Autodesk Inventor part; units mm, degrees
(part 2 of 2)
sketch "スケッチ15" plane through (0, 0, -5) normal (0, 0, -1) x (-1, 0, 0)
  line L0 (-98.885049, -17.626881) -> (-98.885049, -29.356351)
  arc A0 (-98.885049, -29.356351) -> (-98.708578, -29.923625) centre (-97.885049, -29.356351) ccw
  arc A1 (-96.237392, -35.660714) -> (-98.708578, -29.923625) centre (-111.885049, -39.000002) ccw
  arc A2 (-96.237392, -35.660714) -> (-94.615037, -36.216716) centre (-95.259414, -35.452009) ccw
  line L1 (-94.615037, -36.216716) -> (-87.366936, -30.109143)
  arc A3 (-87.366936, -30.109143) -> (-87.246605, -28.700058) centre (-88.011313, -29.344435) ccw
  line L2 (-87.246605, -28.700058) -> (-97.120341, -16.982504)
  arc A4 (-97.120341, -16.982504) -> (-98.885049, -17.626881) centre (-97.885049, -17.626881) ccw
  line L3 (-95.269293, -14.523557) -> (-84.952482, -26.766926)
  arc A5 (-84.952482, -26.766926) -> (-83.543397, -26.887257) centre (-84.187774, -26.122549) ccw
  line L4 (-83.543397, -26.887257) -> (-68.236506, -13.988985)
  arc A6 (-68.236506, -13.988985) -> (-68.451315, -12.321243) centre (-68.880883, -13.224277) ccw
  arc A7 (-70.985635, -10.277156) -> (-68.451315, -12.321243) centre (-65.444342, -6) ccw
  arc A8 (-70.985635, -10.277156) -> (-71.610635, -9.902156) centre (-71.777249, -10.888178) ccw
  arc A9 (-73.833202, -9.125) -> (-71.610635, -9.902156) centre (-70.444342, -3) ccw
  arc A10 (-73.833202, -9.125) -> (-74.317325, -9) centre (-74.317325, -10) ccw
  line L5 (-74.317325, -9) -> (-80.016712, -9)
  arc A11 (-80.016712, -9) -> (-80.500835, -9.125) centre (-80.016712, -10) ccw
  arc A12 (-82.723402, -9.902156) -> (-80.500835, -9.125) centre (-83.889695, -3) ccw
  arc A13 (-82.723402, -9.902156) -> (-83.348402, -10.277156) centre (-82.556788, -10.888178) ccw
  arc A14 (-91.952195, -12.294529) -> (-83.348402, -10.277156) centre (-88.889695, -6) ccw
  arc A15 (-91.952195, -12.294529) -> (-92.827195, -12.294529) centre (-92.389695, -13.193747) ccw
  arc A16 (-94.677724, -12.894282) -> (-92.827195, -12.294529) centre (-95.889695, -6) ccw
  arc A17 (-94.677724, -12.894282) -> (-95.269293, -14.523557) centre (-94.504585, -13.87918) ccw
  line L6 (-57.444342, -3) -> (-54.444342, -3)
  arc A18 (-54.444342, -3) -> (-52.444342, -3) centre (-53.444342, -3) ccw
  line L7 (-52.444342, -3) -> (-49.444342, -3)
  line L8 (-49.444342, -3) -> (-49.444342, -6)
  line L9 (-49.444342, -6) -> (-102.219392, -50.47062)
  arc A19 (-121.057661, -50.868582) -> (-102.219392, -50.47062) centre (-111.885049, -39.000002) ccw
  line L10 (-121.057661, -50.868582) -> (-127.651316, -45.772687)
  line L11 (-127.651316, -45.772687) -> (-119.12697, -45.895985)
  arc A20 (-119.12697, -45.895985) -> (-104.885049, -31.858573) centre (-111.885049, -39.000002) ccw
  line L12 (-104.885049, -31.858573) -> (-104.885049, -3)
  line L13 (-104.885049, -3) -> (-101.889695, -3)
  arc A21 (-101.889695, -3) -> (-99.889695, -3) centre (-100.889695, -3) ccw
  line L14 (-99.889695, -3) -> (-96.889695, -3)
  line L15 (-96.889695, -3) -> (-96.889695, -6)
  arc A22 (-96.889695, -6) -> (-94.889695, -6) centre (-95.889695, -6) ccw
  line L16 (-94.889695, -6) -> (-89.889695, -6)
  arc A23 (-89.889695, -6) -> (-87.889695, -6) centre (-88.889695, -6) ccw
  line L17 (-87.889695, -6) -> (-87.889695, -3)
  line L18 (-87.889695, -3) -> (-84.889695, -3)
  arc A24 (-84.889695, -3) -> (-82.889695, -3) centre (-83.889695, -3) ccw
  line L19 (-82.889695, -3) -> (-71.444342, -3)
  arc A25 (-71.444342, -3) -> (-69.444342, -3) centre (-70.444342, -3) ccw
  line L20 (-69.444342, -3) -> (-66.444342, -3)
  line L21 (-66.444342, -3) -> (-66.444342, -6)
  arc A26 (-66.444342, -6) -> (-64.444342, -6) centre (-65.444342, -6) ccw
  line L22 (-64.444342, -6) -> (-59.444342, -6)
  arc A27 (-59.444342, -6) -> (-57.444342, -6) centre (-58.444342, -6) ccw
  line L23 (-57.444342, -6) -> (-57.444342, -3)
  line L24 (-107.885049, -23.783101) -> (-107.885049, -15.626145)
  arc A28 (-107.885049, -15.626145) -> (-109.702802, -15.050577) centre (-108.885049, -15.626145) ccw
  line L25 (-109.702802, -15.050577) -> (-113.542064, -20.505302)
  arc A29 (-113.542064, -20.505302) -> (-113.299879, -21.898624) centre (-112.72431, -21.08087) ccw
  line L26 (-113.299879, -21.898624) -> (-109.460618, -24.600855)
  arc A30 (-109.460618, -24.600855) -> (-107.885049, -23.783101) centre (-108.885049, -23.783101) ccw
  arc A31 (-123.011027, -34.504158) -> (-123.823452, -37.785703) centre (-111.885049, -39.000002) ccw
  line L27 (-123.823452, -37.785703) -> (-124.225152, -41.735024)
  arc A32 (-124.225152, -41.735024) -> (-123.244748, -42.836111) centre (-123.230285, -41.836215) ccw
  line L28 (-123.244748, -42.836111) -> (-120.427294, -42.876863)
  arc A33 (-120.427294, -42.876863) -> (-119.4653, -41.557305) centre (-120.412831, -41.876968) ccw
  arc A34 (-119.448659, -36.393892) -> (-119.4653, -41.557305) centre (-111.885049, -39.000002) ccw
  arc A35 (-119.448659, -36.393892) -> (-119.818541, -35.250375) centre (-120.39411, -36.068129) ccw
  line L29 (-119.818541, -35.250375) -> (-121.508293, -34.061058)
  arc A36 (-121.508293, -34.061058) -> (-123.011027, -34.504158) centre (-122.083862, -34.878811) ccw
  line L30 (-108.30948, -29.07966) -> (-115.026585, -24.351884)
  arc A37 (-115.026585, -24.351884) -> (-116.419907, -24.594069) centre (-115.602154, -25.169638) ccw
  line L31 (-116.419907, -24.594069) -> (-120.259168, -30.048794)
  arc A38 (-120.259168, -30.048794) -> (-120.016984, -31.442116) centre (-119.441415, -30.624363) ccw
  line L32 (-120.016984, -31.442116) -> (-118.091835, -32.797115)
  arc A39 (-118.091835, -32.797115) -> (-116.890576, -32.759433) centre (-117.516266, -31.979362) ccw
  arc A40 (-109.218382, -31.45753) -> (-116.890576, -32.759433) centre (-111.885049, -39.000002) ccw
  arc A41 (-109.218382, -31.45753) -> (-107.885049, -30.514721) centre (-108.885049, -30.514721) ccw
  line L33 (-107.885049, -30.514721) -> (-107.885049, -29.897414)
  arc A42 (-107.885049, -29.897414) -> (-108.30948, -29.07966) centre (-108.885049, -29.897414) ccw
  circle A43 centre (-111.885049, -39.000002) radius 3
  line L34 (-104.885049, -3) -> (-104.889695, -3)
  line L35 (-104.885049, -31.858573) -> (-104.885049, -3)
  arc A44 (-119.12697, -45.895985) -> (-104.885049, -31.858573) centre (-111.885049, -39.000002) ccw
  line L36 (-127.651316, -45.772687) -> (-119.12697, -45.895985)
  line L37 (-126.808053, -37.482129) -> (-127.651316, -45.772687)
  arc A45 (-124.15135, -30.366471) -> (-126.808053, -37.482129) centre (-111.885049, -39.000002) ccw
  line L38 (-104.889695, -3) -> (-124.15135, -30.366471)
  point P0 (0, 0)
  point P1 (0, 0)
  constraints: 90 point on circle, 78 end point, 46 centre point, 11 horizontal, 10 vertical, 194 other
extrude "押し出し17" cut sketch "スケッチ15" against normal blind 4 contours A4 L2 A3 L1 A2 A1 A0 L0 | A17 A16 A15 A14 A13 A12 A11 L5 A10 A9 A8 A7 A6 L4 A5 L3 | A30 L26 A29 L25 A28 L24 | A36 L29 A35 A34 A33 L28 A32 L27 A31 | A42 L33 A41 A40 A39 L32 A38 L31 A37 L30
sketch "スケッチ16" plane through (0, 0, -5) normal (0, 0, -1) x (-1, 0, 0)
  arc A0 (-82.723402, -9.902156) -> (-80.500835, -9.125) centre (-83.889695, -3) ccw
  arc A1 (-82.723402, -9.902156) -> (-83.348402, -10.277156) centre (-82.556788, -10.888178) ccw
  arc A2 (-91.952195, -12.294529) -> (-83.348402, -10.277156) centre (-88.889695, -6) ccw
  arc A3 (-91.952195, -12.294529) -> (-92.827195, -12.294529) centre (-92.389695, -13.193747) ccw
  arc A4 (-94.677724, -12.894282) -> (-92.827195, -12.294529) centre (-95.889695, -6) ccw
  arc A5 (-94.677724, -12.894282) -> (-95.269293, -14.523557) centre (-94.504585, -13.87918) ccw
  line L0 (-95.269293, -14.523557) -> (-84.952482, -26.766926)
  arc A6 (-84.952482, -26.766926) -> (-83.543397, -26.887257) centre (-84.187774, -26.122549) ccw
  line L1 (-83.543397, -26.887257) -> (-68.236506, -13.988985)
  arc A7 (-68.236506, -13.988985) -> (-68.451315, -12.321243) centre (-68.880883, -13.224277) ccw
  arc A8 (-70.985635, -10.277156) -> (-68.451315, -12.321243) centre (-65.444342, -6) ccw
  arc A9 (-70.985635, -10.277156) -> (-71.610635, -9.902156) centre (-71.777249, -10.888178) ccw
  arc A10 (-73.833202, -9.125) -> (-71.610635, -9.902156) centre (-70.444342, -3) ccw
  arc A11 (-73.833202, -9.125) -> (-74.317325, -9) centre (-74.317325, -10) ccw
  line L2 (-74.317325, -9) -> (-80.016712, -9)
  arc A12 (-80.016712, -9) -> (-80.500835, -9.125) centre (-80.016712, -10) ccw
  line L3 (-94.615037, -36.216716) -> (-87.366936, -30.109143)
  arc A13 (-87.366936, -30.109143) -> (-87.246605, -28.700058) centre (-88.011313, -29.344435) ccw
  line L4 (-87.246605, -28.700058) -> (-97.120341, -16.982504)
  arc A14 (-97.120341, -16.982504) -> (-98.885049, -17.626881) centre (-97.885049, -17.626881) ccw
  line L5 (-98.885049, -17.626881) -> (-98.885049, -29.356351)
  arc A15 (-98.885049, -29.356351) -> (-98.708578, -29.923625) centre (-97.885049, -29.356351) ccw
  arc A16 (-96.237392, -35.660714) -> (-98.708578, -29.923625) centre (-111.885049, -39.000002) ccw
  arc A17 (-96.237392, -35.660714) -> (-94.615037, -36.216716) centre (-95.259414, -35.452009) ccw
  line L6 (-127.651316, -45.772687) -> (-119.12697, -45.895985)
  arc A18 (-119.12697, -45.895985) -> (-104.885049, -31.858573) centre (-111.885049, -39.000002) ccw
  line L7 (-104.885049, -31.858573) -> (-104.885049, -3)
  line L8 (-104.885049, -3) -> (-101.889695, -3)
  arc A19 (-101.889695, -3) -> (-99.889695, -3) centre (-100.889695, -3) ccw
  line L9 (-99.889695, -3) -> (-96.889695, -3)
  line L10 (-96.889695, -3) -> (-96.889695, -6)
  arc A20 (-96.889695, -6) -> (-94.889695, -6) centre (-95.889695, -6) ccw
  line L11 (-94.889695, -6) -> (-89.889695, -6)
  arc A21 (-89.889695, -6) -> (-87.889695, -6) centre (-88.889695, -6) ccw
  line L12 (-87.889695, -6) -> (-87.889695, -3)
  line L13 (-87.889695, -3) -> (-84.889695, -3)
  arc A22 (-84.889695, -3) -> (-82.889695, -3) centre (-83.889695, -3) ccw
  line L14 (-82.889695, -3) -> (-71.444342, -3)
  arc A23 (-71.444342, -3) -> (-69.444342, -3) centre (-70.444342, -3) ccw
  line L15 (-69.444342, -3) -> (-66.444342, -3)
  line L16 (-66.444342, -3) -> (-66.444342, -6)
  arc A24 (-66.444342, -6) -> (-64.444342, -6) centre (-65.444342, -6) ccw
  line L17 (-64.444342, -6) -> (-59.444342, -6)
  arc A25 (-59.444342, -6) -> (-57.444342, -6) centre (-58.444342, -6) ccw
  line L18 (-57.444342, -6) -> (-57.444342, -3)
  line L19 (-57.444342, -3) -> (-54.444342, -3)
  arc A26 (-54.444342, -3) -> (-52.444342, -3) centre (-53.444342, -3) ccw
  line L20 (-52.444342, -3) -> (-49.444342, -3)
  line L21 (-49.444342, -3) -> (-49.444342, -6)
  line L22 (-49.444342, -6) -> (-102.219392, -50.47062)
  arc A27 (-121.057661, -50.868582) -> (-102.219392, -50.47062) centre (-111.885049, -39.000002) ccw
  line L23 (-121.057661, -50.868582) -> (-127.651316, -45.772687)
  line L24 (-84.889695, 0.872983) -> (-84.889695, -6)
  arc A28 (-91.535447, -9) -> (-84.889695, -6) centre (-88.889695, -6) ccw
  line L25 (-91.535447, -9) -> (-93.243944, -9)
  arc A29 (-99.889695, -6) -> (-93.243944, -9) centre (-95.889695, -6) ccw
  line L26 (-99.889695, -6) -> (-99.889695, 0.872983)
  arc A30 (-101.885049, 0.87418) -> (-99.889695, 0.872983) centre (-100.889695, -3) ccw
  line L27 (-101.885049, 0.87418) -> (-101.885049, -30.693378)
  arc A31 (-120.335431, -48.878819) -> (-101.885049, -30.693378) centre (-111.885049, -39.000002) ccw
  line L28 (-120.335431, -48.878819) -> (-118.695646, -48.902538)
  line L29 (-118.695646, -48.902538) -> (-119.223138, -48.494866)
  arc A32 (-119.223138, -48.494866) -> (-104.152524, -48.176497) centre (-111.885049, -39.000002) ccw
  line L30 (-104.152524, -48.176497) -> (-52.444342, -4.604868)
  line L31 (-52.444342, -4.604868) -> (-52.444342, 0.872983)
  arc A33 (-54.444342, 0.872983) -> (-52.444342, 0.872983) centre (-53.444342, -3) ccw
  line L32 (-54.444342, 0.872983) -> (-54.444342, -6)
  arc A34 (-61.090093, -9) -> (-54.444342, -6) centre (-58.444342, -6) ccw
  line L33 (-61.090093, -9) -> (-62.79859, -9)
  arc A35 (-69.444342, -6) -> (-62.79859, -9) centre (-65.444342, -6) ccw
  line L34 (-69.444342, -6) -> (-69.444342, 0.872983)
  arc A36 (-73.090093, -6) -> (-69.444342, 0.872983) centre (-70.444342, -3) ccw
  line L35 (-73.090093, -6) -> (-81.243944, -6)
  arc A37 (-84.889695, 0.872983) -> (-81.243944, -6) centre (-83.889695, -3) ccw
  line L36 (-87.366936, -30.109143) -> (-94.615037, -36.216716)
  line L37 (-94.615037, -36.216716) -> (-98.912059, -39.83758)
  line L38 (-98.885049, -29.356351) -> (-98.885049, -17.626881)
  line L39 (-98.885049, -29.356351) -> (-98.885049, -39.000002)
  line L40 (-87.366936, -30.109143) -> (-94.615037, -36.216716)
  line L41 (-68.236506, -13.988985) -> (-83.543397, -26.887257)
  line L42 (-68.236506, -13.988985) -> (-62.315879, -9)
  arc A38 (-94.677724, -12.894282) -> (-95.269293, -14.523557) centre (-94.504585, -13.87918) ccw
  line L43 (-95.269293, -14.523557) -> (-101.885049, -6.672377)
  line L44 (-98.885049, -17.626881) -> (-98.885049, -6.461415)
  point P0 (0, 0)
  point P1 (-84.980691, -6.848341)
  point P2 (-98.885049, -8.65101)
  point P3 (-98.885049, -10.232596)
  point P4 (-69.353346, -6.848341)
  dimension "d151" = 3
  constraints: 34 end point, 23 point on circle, 10 centre point, 5 collinear, 2 point on line, 21 other
  measures "d151" distance between parallel lines of L14 L35
extrude "押し出し18" cut sketch "スケッチ16" against normal blind 4 contours A1 A2 A3 A4 A5 L43 L44 A29 L25 A28 A37 L35 A36 A35 L33 L42 A7 A8 A9 A10 A11 L2 A12 A0 | A15 A16 A17 L37 A31 L39
fillet "フィレット3" radius 1 11 edges at (62.3159, -9, -3) (62.7986, -9, -3) (69.3533, -6.8483, -3) (73.0901, -6, -3) (81.2439, -6, -3) (84.9807, -6.8483, -3) (91.5354, -9, -3) (93.2439, -9, -3) (98.885, -8.651, -3) (98.885, -10.2326, -3) (98.9121, -39.8376, -3)
sketch "スケッチ17" plane through (0, 0, -5) normal (0, 0, -1) x (-1, 0, 0)
  arc A0 (-98.885049, -37.664486) -> (-97.240672, -38.429194) centre (-97.885049, -37.664486) ccw
  line L0 (-97.240672, -38.429194) -> (-87.366936, -30.109143)
  arc A1 (-87.366936, -30.109143) -> (-87.246605, -28.700058) centre (-88.011313, -29.344435) ccw
  line L1 (-87.246605, -28.700058) -> (-97.120341, -16.982504)
  arc A2 (-97.120341, -16.982504) -> (-98.885049, -17.626881) centre (-97.885049, -17.626881) ccw
  line L2 (-98.885049, -17.626881) -> (-98.885049, -37.664486)
  arc A3 (-96.813663, -9.891823) -> (-97.809362, -11.509155) centre (-97.044655, -10.864778) ccw
  line L3 (-97.809362, -11.509155) -> (-84.952482, -26.766926)
  arc A4 (-84.952482, -26.766926) -> (-83.543397, -26.887257) centre (-84.187774, -26.122549) ccw
  line L4 (-83.543397, -26.887257) -> (-65.532789, -11.710713)
  arc A5 (-65.532789, -11.710713) -> (-66.030602, -9.956804) centre (-66.177167, -10.946005) ccw
  arc A6 (-69.116255, -7.586522) -> (-66.030602, -9.956804) centre (-65.444342, -6) ccw
  arc A7 (-69.116255, -7.586522) -> (-70.116255, -6.986522) centre (-70.034233, -7.983153) ccw
  arc A8 (-72.844342, -6.2) -> (-70.116255, -6.986522) centre (-70.444342, -3) ccw
  arc A9 (-72.844342, -6.2) -> (-73.444342, -6) centre (-73.444342, -7) ccw
  line L5 (-73.444342, -6) -> (-80.889695, -6)
  arc A10 (-80.889695, -6) -> (-81.489695, -6.2) centre (-80.889695, -7) ccw
  arc A11 (-84.217782, -6.986522) -> (-81.489695, -6.2) centre (-83.889695, -3) ccw
  arc A12 (-84.217782, -6.986522) -> (-85.217782, -7.586522) centre (-84.299804, -7.983153) ccw
  arc A13 (-91.289695, -9.2) -> (-85.217782, -7.586522) centre (-88.889695, -6) ccw
  arc A14 (-91.289695, -9.2) -> (-91.889695, -9) centre (-91.889695, -10) ccw
  line L6 (-91.889695, -9) -> (-92.889695, -9)
  arc A15 (-92.889695, -9) -> (-93.489695, -9.2) centre (-92.889695, -10) ccw
  arc A16 (-96.813663, -9.891823) -> (-93.489695, -9.2) centre (-95.889695, -6) ccw
  line L7 (-127.651316, -45.772687) -> (-119.12697, -45.895985)
  arc A17 (-119.12697, -45.895985) -> (-104.885049, -31.858573) centre (-111.885049, -39.000002) ccw
  line L8 (-104.885049, -31.858573) -> (-104.885049, -3)
  line L9 (-104.885049, -3) -> (-101.889695, -3)
  arc A18 (-101.889695, -3) -> (-99.889695, -3) centre (-100.889695, -3) ccw
  line L10 (-99.889695, -3) -> (-96.889695, -3)
  line L11 (-96.889695, -3) -> (-96.889695, -6)
  arc A19 (-96.889695, -6) -> (-94.889695, -6) centre (-95.889695, -6) ccw
  line L12 (-94.889695, -6) -> (-89.889695, -6)
  arc A20 (-89.889695, -6) -> (-87.889695, -6) centre (-88.889695, -6) ccw
  line L13 (-87.889695, -6) -> (-87.889695, -3)
  line L14 (-87.889695, -3) -> (-84.889695, -3)
  arc A21 (-84.889695, -3) -> (-82.889695, -3) centre (-83.889695, -3) ccw
  line L15 (-82.889695, -3) -> (-71.444342, -3)
  arc A22 (-71.444342, -3) -> (-69.444342, -3) centre (-70.444342, -3) ccw
  line L16 (-69.444342, -3) -> (-66.444342, -3)
  line L17 (-66.444342, -3) -> (-66.444342, -6)
  arc A23 (-66.444342, -6) -> (-64.444342, -6) centre (-65.444342, -6) ccw
  line L18 (-64.444342, -6) -> (-59.444342, -6)
  arc A24 (-59.444342, -6) -> (-57.444342, -6) centre (-58.444342, -6) ccw
  line L19 (-57.444342, -6) -> (-57.444342, -3)
  line L20 (-57.444342, -3) -> (-54.444342, -3)
  arc A25 (-54.444342, -3) -> (-52.444342, -3) centre (-53.444342, -3) ccw
  line L21 (-52.444342, -3) -> (-49.444342, -3)
  line L22 (-49.444342, -3) -> (-49.444342, -6)
  line L23 (-49.444342, -6) -> (-102.219392, -50.47062)
  arc A26 (-121.057661, -50.868582) -> (-102.219392, -50.47062) centre (-111.885049, -39.000002) ccw
  line L24 (-121.057661, -50.868582) -> (-127.651316, -45.772687)
  line L25 (-104.796901, -47.411789) -> (-60.016711, -9.677996)
  line L26 (-70.444342, -6) -> (-70.444342, 2)
  arc A27 (-73.444342, -7) -> (-70.444342, 2) centre (-70.444342, -3) ccw
  line L27 (-73.444342, -7) -> (-80.889695, -7)
  arc A28 (-83.889695, 2) -> (-80.889695, -7) centre (-83.889695, -3) ccw
  line L28 (-83.889695, 2) -> (-83.889695, -6)
  arc A29 (-91.889695, -10) -> (-83.889695, -6) centre (-88.889695, -6) ccw
  line L29 (-91.889695, -10) -> (-92.889695, -10)
  arc A30 (-100.885049, -6.215503) -> (-92.889695, -10) centre (-95.889695, -6) ccw
  line L30 (-100.885049, -6.215503) -> (-100.885049, -32.071799)
  line L31 (-61.090093, -9) -> (-62.79859, -9)
  arc A31 (-69.444342, -6) -> (-62.79859, -9) centre (-65.444342, -6) ccw
  line L32 (-69.444342, -6) -> (-69.444342, -6)
  line L33 (-69.444342, -6) -> (-67.79859, -6)
  arc A32 (-73.090093, -6) -> (-67.79859, -6) centre (-70.444342, -3) ccw
  line L34 (-73.090093, -6) -> (-81.243944, -6)
  arc A33 (-86.535447, -6) -> (-81.243944, -6) centre (-83.889695, -3) ccw
  line L35 (-86.535447, -6) -> (-84.889695, -6)
  line L36 (-84.889695, -6) -> (-84.889695, -6)
  arc A34 (-91.535447, -9) -> (-84.889695, -6) centre (-88.889695, -6) ccw
  line L37 (-91.535447, -9) -> (-93.243944, -9)
  arc A35 (-99.889695, -6) -> (-93.243944, -9) centre (-95.889695, -6) ccw
  line L38 (-99.889695, -6) -> (-99.889695, -6)
  line L39 (-99.889695, -6) -> (-98.243944, -6)
  arc A36 (-103.535447, -6) -> (-98.243944, -6) centre (-100.889695, -3) ccw
  line L40 (-103.535447, -6) -> (-101.885049, -6)
  line L41 (-101.885049, -6) -> (-101.885049, -30.693378)
  arc A37 (-120.335431, -48.878819) -> (-101.885049, -30.693378) centre (-111.885049, -39.000002) ccw
  line L42 (-120.335431, -48.878819) -> (-118.695646, -48.902538)
  line L43 (-118.695646, -48.902538) -> (-119.223138, -48.494866)
  arc A38 (-119.223138, -48.494866) -> (-104.152524, -48.176497) centre (-111.885049, -39.000002) ccw
  line L44 (-104.152524, -48.176497) -> (-52.444342, -4.604868)
  line L45 (-52.444342, -4.604868) -> (-52.444342, -6)
  line L46 (-52.444342, -6) -> (-50.79859, -6)
  arc A39 (-56.090093, -6) -> (-50.79859, -6) centre (-53.444342, -3) ccw
  line L47 (-56.090093, -6) -> (-54.444342, -6)
  line L48 (-54.444342, -6) -> (-54.444342, -6)
  arc A40 (-61.090093, -9) -> (-54.444342, -6) centre (-58.444342, -6) ccw
  line L49 (-84.952482, -26.766926) -> (-97.809362, -11.509155)
  line L50 (-84.952482, -26.766926) -> (-76.330152, -36.999387)
  arc A41 (-87.366936, -30.109143) -> (-87.246605, -28.700058) centre (-88.011313, -29.344435) ccw
  line L51 (-87.246605, -28.700058) -> (-79.401691, -38.009929)
  line L52 (-97.120341, -16.982504) -> (-87.246605, -28.700058)
  line L53 (-97.120341, -16.982504) -> (-87.246605, -28.700058)
  line L54 (-97.120341, -16.982504) -> (-109.409195, -2.398832)
  arc A42 (-96.813663, -9.891823) -> (-97.809362, -11.509155) centre (-97.044655, -10.864778) ccw
  line L55 (-97.809362, -11.509155) -> (-106.984949, -0.620123)
  point P0 (0, 0)
  point P1 (-83.019351, -29.06105)
  point P2 (-100.885049, -12.514775)
  point P3 (-99.498849, -42.947413)
  point P4 (-85.313474, -30.994181)
  dimension "d155" = 4
  dimension "d156" = 4
  dimension "d157" = 3
  constraints: 56 end point, 31 point on circle, 14 centre point, 4 collinear, 1 point on line, 34 other
  measures "d155" distance between parallel lines of L23 L25
  measures "d156" distance between parallel lines of L30 L8
  measures "d157" distance between parallel lines of L18 L31
extrude "押し出し19" cut sketch "スケッチ17" against normal blind 4 contours A0 L0 A1 L51 L25 A37 L30 L54 A2 L2 | L50 A4 L4 A5 A31 L31 A40 L25
fillet "フィレット4" radius 1 8 edges at (99.4988, -42.9474, -3) (100.885, -32.0718, -3) (85.3135, -30.9942, -3) (83.0194, -29.061, -3) (60.0167, -9.678, -3) (61.0901, -9, -3) (62.7986, -9, -3) (100.885, -12.5148, -3)
sketch "スケッチ18" plane through (0, 0, 0) normal (0, 0, 1) x (1, 0, 0)
  line L0 (54.444342, -3) -> (57.444342, -3)
  line L1 (57.444342, -3) -> (57.444342, -6)
  arc A0 (57.444342, -6) -> (59.444342, -6) centre (58.444342, -6) ccw
  line L2 (59.444342, -6) -> (64.444342, -6)
  arc A1 (64.444342, -6) -> (66.444342, -6) centre (65.444342, -6) ccw
  line L3 (66.444342, -6) -> (66.444342, -3)
  line L4 (66.444342, -3) -> (69.444342, -3)
  arc A2 (69.444342, -3) -> (71.444342, -3) centre (70.444342, -3) ccw
  line L5 (71.444342, -3) -> (82.889695, -3)
  arc A3 (82.889695, -3) -> (84.889695, -3) centre (83.889695, -3) ccw
  line L6 (84.889695, -3) -> (87.889695, -3)
  line L7 (87.889695, -3) -> (87.889695, -6)
  arc A4 (87.889695, -6) -> (89.889695, -6) centre (88.889695, -6) ccw
  line L8 (89.889695, -6) -> (94.889695, -6)
  arc A5 (94.889695, -6) -> (96.889695, -6) centre (95.889695, -6) ccw
  line L9 (96.889695, -6) -> (96.889695, -3)
  line L10 (96.889695, -3) -> (99.889695, -3)
  arc A6 (99.889695, -3) -> (101.889695, -3) centre (100.889695, -3) ccw
  line L11 (101.889695, -3) -> (104.885049, -3)
  line L12 (104.885049, -3) -> (104.885049, -31.858573)
  arc A7 (104.885049, -31.858573) -> (119.12697, -45.895985) centre (111.885049, -39.000002) ccw
  line L13 (119.12697, -45.895985) -> (127.651316, -45.772687)
  line L14 (127.651316, -45.772687) -> (121.057661, -50.868582)
  arc A8 (102.219392, -50.47062) -> (121.057661, -50.868582) centre (111.885049, -39.000002) ccw
  line L15 (102.219392, -50.47062) -> (49.444342, -6)
  line L16 (49.444342, -6) -> (49.444342, -3)
  line L17 (49.444342, -3) -> (52.444342, -3)
  arc A9 (52.444342, -3) -> (54.444342, -3) centre (53.444342, -3) ccw
  line L18 (99.120341, -14.609024) -> (85.957851, -30.229473)
  arc A10 (85.957851, -30.229473) -> (86.078182, -31.638558) centre (86.722559, -30.87385) ccw
  line L19 (86.078182, -31.638558) -> (97.304324, -41.098208)
  arc A11 (97.304324, -41.098208) -> (98.944155, -40.238251) centre (97.948701, -40.3335) ccw
  arc A12 (100.742192, -32.303978) -> (98.944155, -40.238251) centre (111.885049, -39.000002) ccw
  arc A13 (100.742192, -32.303978) -> (100.885049, -31.788899) centre (99.885049, -31.788899) ccw
  line L20 (100.885049, -31.788899) -> (100.885049, -15.253401)
  arc A14 (100.885049, -15.253401) -> (99.120341, -14.609024) centre (99.885049, -15.253401) ccw
  line L21 (83.663728, -28.296342) -> (97.809362, -11.509155)
  arc A15 (97.809362, -11.509155) -> (96.813663, -9.891823) centre (97.044655, -10.864778) ccw
  arc A16 (93.489695, -9.2) -> (96.813663, -9.891823) centre (95.889695, -6) ccw
  arc A17 (93.489695, -9.2) -> (92.889695, -9) centre (92.889695, -10) ccw
  line L22 (92.889695, -9) -> (91.889695, -9)
  arc A18 (91.889695, -9) -> (91.289695, -9.2) centre (91.889695, -10) ccw
  arc A19 (85.217782, -7.586522) -> (91.289695, -9.2) centre (88.889695, -6) ccw
  arc A20 (85.217782, -7.586522) -> (84.217782, -6.986522) centre (84.299804, -7.983153) ccw
  arc A21 (81.489695, -6.2) -> (84.217782, -6.986522) centre (83.889695, -3) ccw
  arc A22 (81.489695, -6.2) -> (80.889695, -6) centre (80.889695, -7) ccw
  line L23 (80.889695, -6) -> (73.444342, -6)
  arc A23 (73.444342, -6) -> (72.844342, -6.2) centre (73.444342, -7) ccw
  arc A24 (70.116255, -6.986522) -> (72.844342, -6.2) centre (70.444342, -3) ccw
  arc A25 (70.116255, -6.986522) -> (69.116255, -7.586522) centre (70.034233, -7.983153) ccw
  arc A26 (63.044342, -9.2) -> (69.116255, -7.586522) centre (65.444342, -6) ccw
  arc A27 (63.044342, -9.2) -> (62.444342, -9) centre (62.444342, -10) ccw
  line L24 (62.444342, -9) -> (61.950732, -9)
  arc A28 (61.950732, -9) -> (61.306355, -10.764708) centre (61.950732, -10) ccw
  line L25 (61.306355, -10.764708) -> (82.254643, -28.416673)
  arc A29 (82.254643, -28.416673) -> (83.663728, -28.296342) centre (82.89902, -27.651965) ccw
  point P0 (0, 0)
equation "\"d9\" = d7"
equation "\"d26\" = d7"
